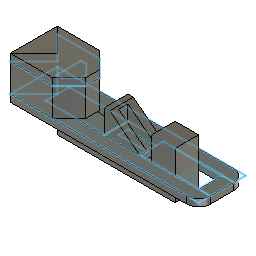
corner-clamp-v1 (Autodesk Fusion 360 design; units mm, degrees)
Autodesk Fusion 360 part; units mm, degrees
sketch "Sketch1" plane through (0, 0, 0) normal (0, 0, 1) x (1, 0, 0) in component "inner-clamp"
  line L0 (-10, 35) -> (70, 35)
  line L1 (70, 35) -> (70, 15)
  line L2 (70, 15) -> (-10, 15)
  line L3 (-10, 15) -> (-10, 35)
  line L4 (25, 30) -> (25, 20)
  line L5 (-10, 15) -> (0, 25)
  line L6 (0, 25) -> (-10, 35)
  line L7 (0, 30) -> (25, 30)
  line L8 (25, 30) -> (25, 20)
  line L9 (25, 20) -> (0, 20)
  line L10 (0, 20) -> (0, 30)
  line L11 (65, 30) -> (40, 30)
  line L12 (40, 30) -> (40, 20)
  line L13 (40, 20) -> (65, 20)
  line L14 (65, 20) -> (65, 30)
  line L15 (25, 30) -> (70, 30)
  line L16 (25, 20) -> (70, 20)
  line L17 (40, 27) -> (28, 27)
  line L18 (28, 27) -> (28, 23)
  line L19 (28, 23) -> (40, 23)
  constraint horizontal L0
  constraint vertical L1
  constraint horizontal L2
  constraint vertical L3
  constraint vertical L4
  constraint perpendicular L5 L6
  constraint horizontal L7
  constraint vertical L8
  constraint horizontal L9
  constraint vertical L10
  constraint horizontal L11
  constraint vertical L12
  constraint horizontal L13
  constraint vertical L14
  constraint coincident L1 L15.end
  constraint perpendicular L1 L15
  constraint coincident L1 L16.end
  constraint perpendicular L1 L16
  constraint coincident L12 L17.start
  constraint perpendicular L12 L17
  constraint perpendicular L17 L18
  constraint coincident L12 L19.end
  constraint perpendicular L12 L19
extrude "Extrude3" add sketch "Sketch1" along normal blind 10 contours L4 L8 L12 L15 L16 L17 L18 L19 makes body 1 in component "inner-clamp"
extrude "Extrude2" add sketch "Sketch1" along normal blind 15 separate body contours L3 L5 L6 makes body 2 in component "inner-clamp"
extrude "Extrude1" add sketch "Sketch1" against normal blind 3 separate body contours L3 L5 L6 | L0 L1 L6 L7 L10 L11 L15 | L1 L2 L5 L9 L10 L13 L16 | L1 L14 L15 L16 | L4 L8 L12 L15 L16 L17 L18 L19 | L12 L17 L18 L19 makes body 3 in component "inner-clamp"
fillet "Fillet1" radius 5 2 edges at (70, 15, -1.5) (70, 35, -1.5) on bodies 3 in component "inner-clamp"
sketch "Sketch2" plane through (0, 30, 0) normal (0, -1, 0) x (1, 0, 0) in component "outer-clamp-slider"
  line L0 (25, 0) -> (0, 0)
  line L1 (0, 0) -> (0, -3)
  line L2 (0, -3) -> (25, -3)
  line L3 (25, -3) -> (25, 0)
  line L4 (5, 12) -> (5, -10)
  line L5 (5, -10) -> (55, -10)
  line L6 (55, -10) -> (55, 10)
  line L7 (55, 10) -> (45, 10)
  line L8 (45, 10) -> (45, -3)
  line L9 (45, -3) -> (11, -3)
  line L10 (11, -3) -> (11, 12)
  line L11 (11, 12) -> (5, 12)
  constraint perpendicular L2 L4
  constraint perpendicular L4 L5
  constraint perpendicular L5 L6
  constraint perpendicular L6 L7
  constraint perpendicular L5 L8
  constraint coincident L2 L9.end
  constraint perpendicular L8 L9
  constraint perpendicular L2 L10
  constraint perpendicular L4 L11
extrude "Extrude1'" add sketch "Sketch2" along normal blind 10 separate body contours L0 L2 L4 L10 | L0 L4 L10 L11 | L2 L4 L5 L6 L7 L8 L9 makes body 4 in component "outer-clamp-slider"
chamfer "Chamfer1" distance 4 angle 45 2 edges at (11, 20, 4.5) (11, 30, 4.5) on bodies 4 in component "outer-clamp-slider"
sketch "Sketch1 (2)" plane through (0, 0, 12) normal (0, 0, 1) x (-1, 0, 0) in component "outer-clamp"
  line L0 (-11, -26) -> (-7, -30)
  line L1 (-7, -30) -> (-5, -30)
  line L2 (-5, -30) -> (-5, -20)
  line L3 (-5, -20) -> (-7, -20)
  line L4 (-7, -20) -> (-11, -24)
  line L5 (-11, -24) -> (-11, -26)
  line L6 (-4.8, -19.8) -> (-7.1, -19.8)
  line L7 (-7.1, -19.8) -> (-11.2, -23.9)
  line L8 (-11.2, -23.9) -> (-11.2, -26.05)
  line L9 (-11.2, -26.05) -> (-7.05, -30.2)
  line L10 (-7.05, -30.2) -> (-4.8, -30.2)
  line L11 (-4.8, -30.2) -> (-4.8, -19.8)
  line L12 (0, -25) -> (10, -35)
  line L13 (10, -35) -> (-8, -35)
  line L14 (-8, -35) -> (-15, -28)
  line L15 (-15, -28) -> (-15, -22)
  line L16 (-15, -22) -> (-8, -15)
  line L17 (-8, -15) -> (10, -15)
  line L18 (10, -15) -> (0, -25)
  constraint parallel L0 L9
  constraint perpendicular L5 L10
  constraint perpendicular L10 L11
  constraint horizontal L13
  constraint parallel L12 L14
  constraint vertical L15
  constraint perpendicular L12 L16
  constraint horizontal L17
  constraint perpendicular L12 L18
extrude "Extrude2'" add sketch "Sketch1 (2)" along normal blind 3 separate body contours L0 L1 L2 L3 L4 L5 | L6 L7 L8 L9 L10 L11 | L12 L13 L14 L15 L16 L17 L18 makes body 5 in component "outer-clamp"
extrude "Extrude1''" add sketch "Sketch1 (2)" against normal blind 12 separate body contours L12 L13 L14 L15 L16 L17 L18 makes body 6 in component "outer-clamp"
sketch "Sketch2 (2)" plane through (0, 20, 0) normal (0, -1, 0) x (1, 0, 0) in component "inner-clamp"
  line L0 (25, 0) -> (40, 0)
  line L1 (40, 0) -> (40, 10)
  line L2 (40, 10) -> (25, 10)
  line L3 (25, 10) -> (25, 0)
  line L4 (40, 0) -> (26, 11)
  constraint coincident L0.end L1.start
extrude "Extrude4" cut sketch "Sketch2 (2)" against normal blind 10 contours L1 L2 L4 bodies 1 in component "inner-clamp"
component "outer-clamp-slider" placed x (1, 0, 0) y (0, 1, 0) z (0, 0, 1) at (0, 0, 0)
component "inner-clamp" placed x (1, 0, 0) y (0, 1, 0) z (0, 0, 1) at (0, 0, 0)
component "outer-clamp" placed x (1, 0, 0) y (0, 1, 0) z (0, 0, 1) at (0, 0, 0)
